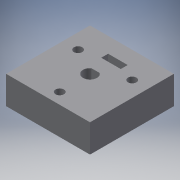
# Autodesk Inventor part: Фланец
Saved by Autodesk Inventor 2018.3 (Build 223284000, 284)
## iProperties
Created: 2018-06-16
Part Number: Фланец
Material: Типовые
Document SubType Name: Modeling
Designer: Leancher
Density: 1 g/cm^3
Appearance: По умолчанию
Author: Leancher
Autodesk Inventor part; units mm, degrees
ref_plane "YZ Plane" through (0, 0, 0) normal (1, 0, 0) x (0, 1, 0)
ref_plane "XZ Plane" through (0, 0, 0) normal (0, 1, 0) x (-1, 0, 0)
ref_plane "XY Plane" through (0, 0, 0) normal (0, 0, 1) x (1, 0, 0)
ref_plane "РабПлоскость2" through (0, 0, 0) normal (0, 0, 1) x (1, 0, 0)
sketch "Эскиз1" plane through (0, 0, 0) normal (0, 0, 1) x (1, 0, 0)
  line L0 (-1.5, 2) -> (1.5, 2)
  arc A0 (-1.5, 2) -> (1.5, 2) centre (0, 0) ccw
  line L1 (-15, 0) -> (-15, 15)
  line L2 (-15, 15) -> (0, 15)
  line L3 (-15, 0) -> (-15, -15)
  line L4 (-15, -15) -> (15, -15)
  line L5 (15, -15) -> (15, 15)
  line L6 (15, 15) -> (0, 15)
  circle A1 centre (-9.6106, 5.3514) radius 1.5
  circle A2 centre (0.1709, -10.9987) radius 1.5
  circle A3 centre (9.4397, 5.6473) radius 1.5
  line L7 (0, 7) -> (4, 7)
  line L8 (4, 7) -> (4, 9.4684)
  line L9 (4, 9.4684) -> (-2.9796, 9.4684)
  line L10 (-2.9796, 9.4684) -> (-2.9796, 7)
  line L11 (-2.9796, 7) -> (0, 7)
  dimension "d1" = 15
  dimension "d2" = 15
  dimension "d3" = 15
  dimension "d4" = 30
  dimension "d6" = 3
  dimension "d9" = 3
  dimension "d10" = 3
  dimension "d13" = 4
  constraints: 24 end point, 7 perpendicular, 4 centre point, 2 point on circle, 1 point on line, 1 vertical
  measures "d1" distance of L1.end L2.end
  measures "d2" distance of L1.start L1.end
  measures "d3" distance of L1.start L3.end
  measures "d4" distance of L3.end L4.end
  measures "d6" diameter of A1
  measures "d9" diameter of A2
  measures "d10" diameter of A3
  measures "d13" distance of L7.start L7.end
extrude "Выдавливание1" add sketch "Эскиз1" along normal blind 10
